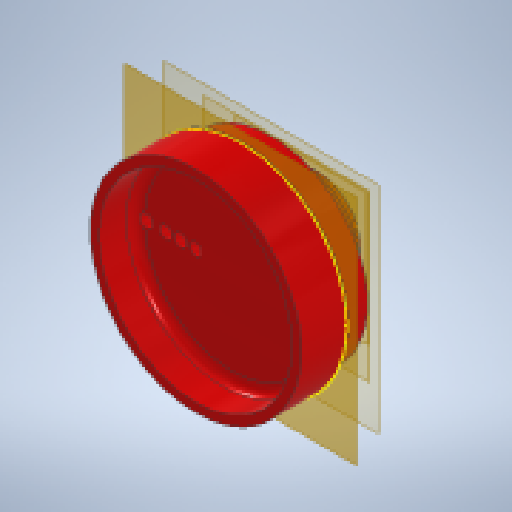
# Autodesk Inventor part: GrundkörperGegenstück
Saved by Autodesk Inventor 2024 (Build 280153000, 153)
## iProperties
Created: 2024-03-18
Part Number: GrundkörperGegenstück
Material: Generic
Document SubType Name: Modeling
Designer: Daniel Nussbaum
Density: 1 g/cm^3
Appearance: Default
Author: Daniel Nussbaum
Autodesk Inventor part; units mm, degrees
ref_plane "Work Plane1" through (-2.5, 0, -10) normal (0, 0, 1) x (1, 0, 0)
sketch "Sketch2" plane through (-2.5, 0, -10) normal (0, 0, 1) x (1, 0, 0)
  circle A0 centre (-32.5, 0) radius 32
  circle A1 centre (-32.5, 0) radius 25 projected
  point P0 (2.5, 0)
  constraints: 1 centre point
ref_plane "Work Plane3" through (-10, 0, -15) normal (0, 0, 1) x (1, 0, 0)
sketch "Sketch3" plane through (-10, 0, -15) normal (0, 0, 1) x (1, 0, 0)
  circle A0 centre (-25, 0) radius 24.5
  circle A1 centre (-25, 0) radius 20 projected
  point P0 (10, 0)
  constraints: 1 centre point
ref_plane "Work Plane5" through (-15, 0, -20) normal (0, 0, 1) x (1, 0, 0)
sketch "Sketch4" plane through (-15, 0, -20) normal (0, 0, 1) x (1, 0, 0)
  circle A0 centre (-20, 0) radius 19.5
  circle A1 centre (-20, 0) radius 15 projected
  point P0 (15, 0)
  constraints: 1 centre point
ref_plane "Work Plane7" through (-20, 0, -25) normal (0, 0, 1) x (1, 0, 0)
sketch "Sketch5" plane through (-20, 0, -25) normal (0, 0, 1) x (1, 0, 0)
  arc A0 (-29.4575, -1.1094) -> (-29.4575, 1.1094) centre (-15, 0) ccw
  arc A1 (-29.4575, 1.1094) -> (-29.4575, -1.1094) centre (-15, 0) ccw
  point P0 (20, 0)
  constraints: 4 point on circle, 2 centre point
ref_plane "Work Plane8" through (0, 0, 0) normal (0, 0, 1) x (1, 0, 0)
sketch "Sketch7" plane through (0, 0, 0) normal (0, 0, 1) x (1, 0, 0)
  circle A0 centre (-35, 0) radius 35 projected
  circle A1 centre (-35, 0) radius 32.5 projected
  point P0 (0, 0)
  constraints: 1 horizontal alignment
ref_plane "Work Plane9" through (-70, -35, 0) normal (0, 0, 1) x (1, 0, 0)
extrude "Extrusion6" add sketch "Sketch2" along normal up to surface (10 mm away)
ref_plane "Work Plane10" through (-70, -35, 0) normal (0, 0, 1) x (1, 0, 0)
extrude "Extrusion7" add sketch "Sketch3" along normal up to surface (15 mm away)
ref_plane "Work Plane11" through (-70, -35, 0) normal (0, 0, 1) x (1, 0, 0)
extrude "Extrusion8" add sketch "Sketch4" along normal up to surface (20 mm away)
ref_plane "Work Plane12" through (-70, -35, 0) normal (0, 0, 1) x (1, 0, 0)
extrude "Extrusion9" add sketch "Sketch5" along normal up to surface (25 mm away)
ref_plane "Work Plane13" through (0, 0, 0) normal (0, 0, 1) x (1, 0, 0)
sketch "Sketch8" plane through (0, 0, 0) normal (0, 0, 1) x (1, 0, 0)
  circle A0 centre (-35, 0) radius 25 projected
  circle A1 centre (-35, 0) radius 32 projected
  circle A2 centre (-35, 0) radius 20 projected
  circle A3 centre (-35, 0) radius 24.5 projected
  circle A4 centre (-35, 0) radius 15 projected
  circle A5 centre (-35, 0) radius 19.5 projected
  circle A6 centre (-35, 0) radius 14.5 projected
  circle A7 centre (-35, 0) radius 35 projected
  circle A8 centre (-35, 0) radius 32.5 projected
  point P0 (0, 0)
  constraints: 1 horizontal alignment
ref_plane "Work Plane14" through (-67.5, -32.5, -10) normal (0, 0, 1) x (1, 0, 0)
extrude "Extrusion10" add sketch "Sketch8" against normal up to surface (10 mm away) contours A0 | A2 | A3 | A4 | A5 | A6
ref_plane "Work Plane15" through (-60, -25, -15) normal (0, 0, 1) x (1, 0, 0)
extrude "Extrusion11" add sketch "Sketch8" against normal up to surface (15 mm away) contours A2 | A4 | A5 | A6
ref_plane "Work Plane16" through (-55, -20, -20) normal (0, 0, 1) x (1, 0, 0)
extrude "Extrusion12" add sketch "Sketch8" against normal up to surface (20 mm away) contours A4 | A6
ref_plane "Work Plane17" through (0, 0, 0) normal (0, 0, 1) x (1, 0, 0)
ref_plane "Work Plane18" through (0, 0, 0) normal (0, 0, 1) x (1, 0, 0)
sketch "Sketch10" plane through (0, 0, 0) normal (0, 0, 1) x (1, 0, 0)
  circle A0 centre (-35, 0) radius 35 projected
  circle A1 centre (-35, 0) radius 32.5 projected
  circle A2 centre (-35, 0) radius 32 projected
  point P0 (0, 0)
  constraints: 1 horizontal alignment
extrude "Extrusion13" add sketch "Sketch10" along normal blind 15 contours A0 | A1 | A2
sketch "Sketch11" plane through (-35, 0, 15) normal (0, 0, 1) x (1, 0, 0)
  circle A0 centre (0, 0) radius 35 projected
  circle A1 centre (0, 0) radius 32 projected
  circle A2 centre (0, 0) radius 24.5 projected
  circle A3 centre (0, 0) radius 32 projected
  circle A4 centre (0, 0) radius 19.5 projected
  circle A5 centre (0, 0) radius 24.5 projected
  circle A6 centre (0, 0) radius 14.5 projected
  circle A7 centre (0, 0) radius 19.5 projected
  circle A8 centre (0, 0) radius 14.5 projected
  point P0 (35, 0)
extrude "Extrusion14" cut sketch "Sketch11" against normal blind 12 contours A1 | A2 | A4 | A6
sketch "Sketch12" plane through (-35, 0, 3) normal (0, 0, 1) x (1, 0, 0)
  circle A0 centre (0, 0) radius 24.5 projected
  circle A1 centre (0, 0) radius 32 projected
  circle A2 centre (0, 0) radius 19.5 projected
  circle A3 centre (0, 0) radius 24.5 projected
  circle A4 centre (0, 0) radius 14.5 projected
  circle A5 centre (0, 0) radius 19.5 projected
  circle A6 centre (0, 0) radius 14.5 projected
  line L0 (-32, 0) -> (-24.5, 0)
  line L1 (-24.5, 0) -> (-19.5, 0)
  line L2 (-19.5, 0) -> (-14.5, 0)
  line L3 (-14.5, 0) -> (0, 0)
  circle A7 centre (-17, 0) radius 2
  circle A8 centre (-22, 0) radius 2
  circle A9 centre (-28.25, 0) radius 2
  line L4 (-14.5, 0) -> (-14.5, 3.413)
  circle A10 centre (-12, 0) radius 2
  point P0 (35, 0)
  dimension "d34" = 4
  dimension "d35" = 4
  dimension "d36" = 4
  constraints: 10 end point, 4 centre point, 4 horizontal, 4 horizontal alignment, 3 midpoint, 1 symmetric about line, 1 vertical, 5 other
  measures "d34" diameter of A7
  measures "d35" diameter of A8
  measures "d36" diameter of A9
hole "Hole1" at (-63.25, 0, 3) at (-57, 0, 3) at (-52, 0, 3) at (-47, 0, 3) direction (0, 0, -1) diameter 4 end through all
fillet "Fillet1" radius 3 1 edges at (-67, 0, 3)
sketch "Sketch14" plane through (-35, 0, 0) normal (0, 0, -1) x (-1, 0, 0)
  circle A0 centre (0, 0) radius 35 projected
  circle A1 centre (0, 0) radius 32 projected
  point P0 (-35, 0)
extrude "Extrusion15" add sketch "Sketch14" along normal blind 0.5
body "Solid2"
